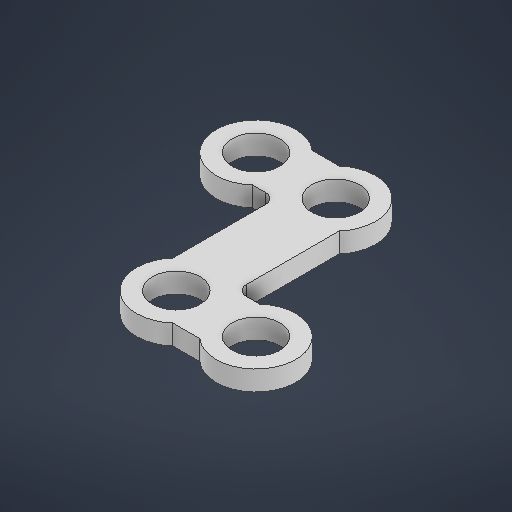
# Autodesk Inventor part: lin-2-turn-4lab-8w
Saved by Autodesk Inventor 2025.4 (Build 294407000, 407)
## iProperties
Created: 2026-09-15
Part Number: lin-2-turn-4lab-8w
Material: Generic
Document SubType Name: Modeling
Designer: User
Density: 1 g/cm^3
Appearance: Default
Author: User
Autodesk Inventor part; units mm, degrees
ref_plane "YZ Plane" through (0, 0, 0) normal (1, 0, 0) x (0, 1, 0)
ref_plane "XZ Plane" through (0, 0, 0) normal (0, 1, 0) x (-1, 0, 0)
ref_plane "XY Plane" through (0, 0, 0) normal (0, 0, 1) x (1, 0, 0)
sketch "Sketch1" plane through (0, 0, 0) normal (0, 1, 0) x (-1, 0, 0)
  line L0 (-1.5, -4) -> (1.5, -4)
  line L1 (1.5, -2) -> (1.5, 4)
  line L2 (1.5, 4) -> (-1.5, 4)
  line L3 (-1.5, 2) -> (-1.5, -4)
  line L4 (-1.5, -4) -> (1.5, 4) construction
  line L5 (1.5, -4) -> (-1.5, 4) construction
  circle A0 centre (0, 4) radius 1.2
  circle A1 centre (0, -4) radius 1.2
  circle A2 centre (0, -4) radius 2
  circle A3 centre (0, 4) radius 2
  line L6 (-2, 2.5) -> (-4, 2.5)
  line L7 (-4, 2.5) -> (-4, 5.5)
  line L8 (-4, 5.5) -> (0, 5.5)
  line L9 (0, 5.5) -> (0, 2.5)
  line L10 (2, -2.5) -> (4, -2.5)
  line L11 (4, -2.5) -> (4, -5.5)
  line L12 (4, -5.5) -> (0, -5.5)
  line L13 (0, -5.5) -> (0, -2.5)
  circle A4 centre (4, -4) radius 1.2
  circle A5 centre (4, -4) radius 2
  circle A6 centre (-4, 4) radius 1.2
  circle A7 centre (-4, 4) radius 2
  arc A8 (-1.5, 2) -> (-2, 2.5) centre (-2, 2) ccw
  arc A9 (1.5, -2) -> (2, -2.5) centre (2, -2) ccw
  point P0 (0, 0)
  point P1 (-1.5, -2.6771)
  point P2 (1.5, -2.6771)
  point P3 (1.5, 2.6771)
  point P4 (-1.5, 2.6771)
  point P5 (-2.6771, 2.5)
  point P6 (-1.5, 2.5)
  point P7 (-1.3229, 5.5)
  point P8 (-2.6771, 5.5)
  point P9 (2.6771, -5.5)
  point P10 (2.6771, -2.5)
  point P11 (1.5, -2.5)
  point P12 (1.3229, -5.5)
  point P13 (-4, 5.2)
  point P14 (-4, 2.8)
  point P15 (4, -5.2)
  point P16 (4, -2.8)
  dimension "d0" = 3
  dimension "linkPitchWidth" = 8
  dimension "d3" = 2.4
  dimension "d4" = 4
  dimension "linkPitchLengthB" = 4
  dimension "d9" = 3
  dimension "linkPitchLengthA" = 4
  dimension "d11" = 3
  dimension "d12" = 0.5
  constraints: 28 end point, 10 centre point, 8 midpoint, 7 equal radius, 6 parallel, 4 coincident, 4 point on circle, 4 point on line, 4 tangent, 3 horizontal, 3 perpendicular
  measures "d0" distance of L2.end L1.end
  measures "linkPitchWidth" distance of L1.end L0.end
  measures "d3" diameter of A1
  measures "d4" diameter of A2
  measures "linkPitchLengthB" distance of L7.end L8.end
  measures "d9" distance of L6.end L7.end
  measures "linkPitchLengthA" distance of L11.end L12.end
  measures "d11" distance of L10.end L11.end
  measures "d12" radius of A8
extrude "Extrusion1" add sketch "Sketch1" along normal blind 1 contours L3 A2 L12 L13 A1 L0 | L0 A1 L13 L12 A2 L3 | L3 A8 L6 A7 A3 L1 A9 L10 A5 A2 | A5 L12 A2 | A5 L10 L11 A4 L12 | A5 L12 L11 A4 L10 | A7 L8 L7 A6 L6 | L6 L7 A6 L8 A7 | L8 A3 A7 | A3 L8 L9 A0 L2 L1 | A3 L1 L2 A0 L9 L8
sketch "Sketch2" plane through (0, 1, 0) normal (0, 1, 0) x (1, 0, 0)
  line L0 (2.6771, -2.5) -> (2, -2.5) projected
  arc A0 (1.5, -2) -> (2, -2.5) centre (2, -2) ccw projected
  line L1 (1.5, -2) -> (1.5, 2.6771) projected
  arc A1 (1.5, 2.6771) -> (-1.3229, 5.5) centre (0, 4) ccw projected
  line L2 (-1.3229, 5.5) -> (-2.6771, 5.5) projected
  arc A2 (-2.6771, 5.5) -> (-2.6771, 2.5) centre (-4, 4) ccw projected
  line L3 (-2.6771, 2.5) -> (-2, 2.5) projected
  arc A3 (-1.5, 2) -> (-2, 2.5) centre (-2, 2) ccw projected
  line L4 (-1.5, 2) -> (-1.5, -2.6771) projected
  arc A4 (-1.5, -2.6771) -> (1.3229, -5.5) centre (0, -4) ccw projected
  line L5 (1.3229, -5.5) -> (2.6771, -5.5) projected
  arc A5 (2.6771, -5.5) -> (2.6771, -2.5) centre (4, -4) ccw projected
  circle A6 centre (4, -4) radius 1.2 projected
  circle A7 centre (0, -4) radius 1.2 projected
  circle A8 centre (0, 4) radius 1.2 projected
  circle A9 centre (-4, 4) radius 1.2 projected
  point P0 (0, 0)
extrude "Extrusion2" [suppressed]
sketch "Sketch3" plane through (0, 1, 0) normal (0, 1, 0) x (1, 0, 0)
  line L0 (2.6771, -2.5) -> (2, -2.5) projected
  arc A0 (1.5, -2) -> (2, -2.5) centre (2, -2) ccw projected
  line L1 (1.5, -2) -> (1.5, 2.6771) projected
  arc A1 (1.5, 2.6771) -> (-1.3229, 5.5) centre (0, 4) ccw projected
  line L2 (-1.3229, 5.5) -> (-2.6771, 5.5) projected
  arc A2 (-2.6771, 5.5) -> (-2.6771, 2.5) centre (-4, 4) ccw projected
  line L3 (-2.6771, 2.5) -> (-2, 2.5) projected
  arc A3 (-1.5, 2) -> (-2, 2.5) centre (-2, 2) ccw projected
  line L4 (-1.5, 2) -> (-1.5, -2.6771) projected
  arc A4 (-1.5, -2.6771) -> (1.3229, -5.5) centre (0, -4) ccw projected
  line L5 (1.3229, -5.5) -> (2.6771, -5.5) projected
  arc A5 (2.6771, -5.5) -> (2.6771, -2.5) centre (4, -4) ccw projected
  circle A6 centre (4, -4) radius 1.2 projected
  circle A7 centre (0, -4) radius 1.2 projected
  circle A8 centre (0, 4) radius 1.2 projected
  circle A9 centre (-4, 4) radius 1.2 projected
  point P0 (0, 0)
extrude "Extrusion3" [suppressed]
body "Solid1"
